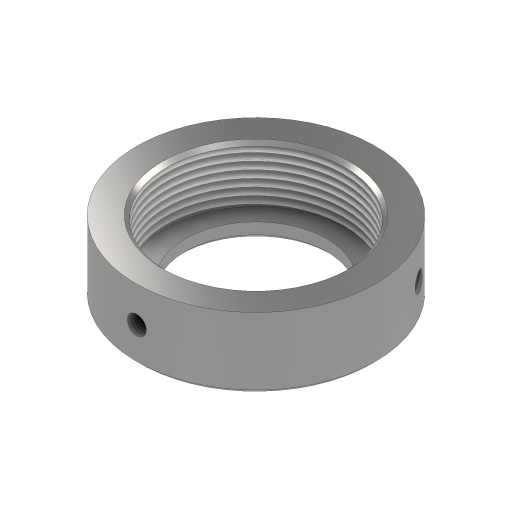
# Autodesk Inventor part: Oring_M48-2_nut
Saved by Autodesk Inventor 2024.2 (Build 282272000, 272)
## iProperties
Created: 2022-12-02
Part Number: Oring_M48-2_nut
Material: Stainless Steel, 440C
Document SubType Name: Modeling
Designer: kuzmin
Density: 7.75 g/cm^3
Appearance: Semi-Polished
Author: kuzmin
Autodesk Inventor part; units mm, degrees
ref_plane "YZ Plane" through (0, 0, 0) normal (1, 0, 0) x (0, 1, 0)
ref_plane "XZ Plane" through (0, 0, 0) normal (0, 1, 0) x (-1, 0, 0)
sketch "Sketch1" plane through (0, 0, 0) normal (0, 0, 1) x (1, 0, 0)
  line L0 (19, 0) -> (32, 0)
  line L1 (32, 0) -> (32, 19)
  line L2 (32, 19) -> (24, 19)
  line L3 (24, 19) -> (24, 4)
  line L4 (24, 4) -> (19, 4)
  line L5 (19, 4) -> (19, 0)
  line L6 (0, 0) -> (0, 12.2084)
  dimension "d0" = 48
  dimension "d1" = 15
  dimension "d2" = 4
  dimension "d4" = 8
  dimension "d17" = 38
  constraints: 14 end point, 5 perpendicular, 1 horizontal, 1 horizontal alignment
  measures "d0" diameter of L3 L6
  measures "d1" distance of L2.end L3.end
  measures "d2" distance of L4.end L0.start
  measures "d4" distance of L1.end L2.end
  measures "d17" diameter of L5 L6
revolve "Revolution1" add sketch "Sketch1" angle 360 about axis through (0, 0, 0) along (0, 1, 0)
chamfer "Chamfer1" distance 1 angle 45 1 edges at (-32, 0, 0)
chamfer "Chamfer2" distance 1 angle 45 1 edges at (-19, 0, 0)
chamfer "Chamfer3" distance 1 angle 45 1 edges at (-24, 19, 0)
thread "Thread1" size "M48x2" class "6H" standard "ANSI Metric M Profile" full length
ref_plane "Work Plane1" through (0, 9.5, 32) normal (0, 0, 1) x (1, 0, 0)
sketch "Sketch3" plane through (0, 9.5, 32) normal (0, 0, 1) x (1, 0, 0)
  circle A0 centre (0, 0) radius 2.5
  point P0 (0, -9.5)
  dimension "d18" = 5
  constraints: 1 centre point
  measures "d18" diameter of A0
extrude "Extrusion1" cut sketch "Sketch3" against normal blind 5
thread "Thread2" size "M5x0.8" class "6H" standard "ANSI Metric M Profile" full length
pattern_circular "Circular Pattern1" count 3 over 360 about axis through (0, 9.5, 0) along (0, 1, 0) of "Extrusion1"
body "Solid1"
